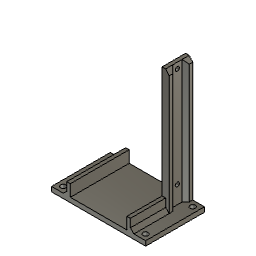
NUC_Mount (Autodesk Fusion 360 design; units mm, degrees)
Autodesk Fusion 360 part; units mm, degrees
sketch "Sketch1" plane through (0, 0, 0) normal (0, 1, 0) x (1, 0, 0)
  line L0 (0, 0) -> (-48, 0) construction
  line L1 (-48, 0) -> (-48, -115) construction
  line L2 (-48, -115) -> (0, -115) construction
  line L3 (0, -115) -> (0, 0) construction
  line L4 (0, -105) -> (3, -105)
  line L5 (3, -105) -> (3, 0)
  line L6 (3, 0) -> (16, 0)
  line L7 (16, 0) -> (16, 4)
  line L8 (16, 4) -> (-64, 4)
  line L9 (-64, 4) -> (-64, 0)
  line L10 (-64, 0) -> (-51, 0)
  line L11 (-51, 0) -> (-51, -10)
  line L12 (-51, -10) -> (-48, -10)
  line L13 (-48, -10) -> (-48, 0)
  line L14 (-48, 0) -> (0, 0)
  line L15 (0, 0) -> (0, -105)
  line L16 (0, -100) -> (3, -100) construction
  line L17 (3, -15) -> (0, -14.9007) construction
  line L18 (-51, 0) -> (-48, 0)
  line L19 (0, 0) -> (3, 0)
  line L20 (3, -105) -> (6, -101.4247)
  line L21 (6, -101.4247) -> (6, 0)
  line L22 (0, -10) -> (3, -10)
  dimension "d1" = 48
  dimension "d2" = 115
  dimension "d3" = 3
  dimension "d4" = 4
  dimension "d6" = 13
  dimension "d7" = 13
  dimension "d8" = 10
  dimension "d9" = 15
  dimension "d10" = 85
  dimension "d11" = 5
  dimension "d16" = 3
  dimension "d17" = 140
  constraint horizontal L0
  constraint vertical L1
  constraint horizontal L2
  constraint vertical L3
  constraint coincident L0.start L3.end
  constraint coincident L3 L4.start
  constraint perpendicular L3 L4
  constraint perpendicular L4 L5
  constraint perpendicular L3 L6
  constraint perpendicular L6 L7
  constraint perpendicular L7 L8
  constraint perpendicular L8 L9
  constraint perpendicular L9 L10
  constraint perpendicular L8 L11
  constraint coincident L1 L12.end
  constraint perpendicular L1 L12
  constraint perpendicular L3 L14
  constraint equal L7 L9
  constraint coincident L3 L16.start
  constraint coincident L5 L16.end
  constraint perpendicular L5 L16
  constraint coincident L5 L17.start
  constraint coincident L3 L17.end
  constraint coincident L6 L0.start
  constraint equal L4 L12
  constraint coincident L5 L4.end
  constraint vertical L21
  constraint coincident L6 L21.end
  constraint coincident L3 L22.start
  constraint coincident L5 L22.end
  constraint perpendicular L5 L22
  constraint collinear L12 L22
  constraint coincident L4.end L5.start
  measures "d1" distance of L0.start L0.end
  measures "d2" distance of L0.end L1.end
  measures "d3" distance of L4.start L4.end
  measures "d4" distance of L6.end L7.end
  measures "d6" distance of L5.end L6.end
  measures "d7" distance of L9.end L10.end
  measures "d8" distance of L10.end L11.end
  measures "d9" vertical distance of L0.start L17.start
  measures "d10" distance of L16.end L17.start
  measures "d11" distance of L4.end L16.end
  measures "d16" distance of L5 L21
  measures "d17" angle of L20 L21
extrude "Extrude1" add sketch "Sketch1" along normal blind 20 contours L4 L5 L15 L22 | L5 L15 L19 L22 | L6 L7 L8 L9 L10 L14 L18 L19 | L11 L12 L13 L18
extrude "Extrude2" add sketch "Sketch1" against normal blind 30 contours L6 L7 L8 L9 L10 L14 L18 L19
extrude "Extrude3" add sketch "Sketch1" against normal blind 30 contours L5 L15 L19 L22 | L11 L12 L13 L18
sketch "Sketch2" plane through (3, 0, 0) normal (1, 0, 0) x (0, 1, 0)
  line L0 (0, 105) -> (0, 10)
  line L1 (0, 10) -> (-30, 10)
  line L2 (-30, 10) -> (-30, 0)
  line L3 (-30, 0) -> (20, 0)
  line L4 (20, 0) -> (20, 105)
  line L5 (20, 105) -> (0, 105)
  line L6 (10, 105) -> (10, 0) construction
  circle A0 centre (10, 15) radius 1.75
  circle A1 centre (10, 100) radius 1.75
  dimension "d21" = 15
  dimension "d22" = 85
  dimension "d23" = 3.5
  constraint midpoint L5 L6.start
  constraint coincident L3 L6.end
  constraint perpendicular L3 L6
  constraint coincident L6 A0.centre
  constraint coincident L6 A1.centre
  constraint equal A0 A1
  measures "d21" distance of L6.end A0.centre
  measures "d22" distance of A0.centre A1.centre
  measures "d23" diameter of A0
extrude "Extrude4" cut sketch "Sketch2" against normal blind 12 contours A0 | A1
extrude "Extrude5" add sketch "Sketch1" along normal blind 3 contours L5 L6 L20 L21
chamfer "Chamfer1" distance 3 angle 45 1 edges at (3, 3, 52.5)
chamfer "Chamfer2" distance 3 angle 45 1 edges at (3, -15, 0)
chamfer "Chamfer3" distance 3 angle 45 1 edges at (-51, -5, 0)
extrude "Extrude6" add sketch "Sketch1" against normal blind 3 from surface at 20 contours L5 L6 L20 L21
chamfer "Chamfer4" distance 3 angle 45 1 edges at (3, 17, 52.5)
sketch "Sketch3" plane through (0, 0, 0) normal (0, 0, 1) x (1, 0, 0)
  line L0 (11, -25) -> (-59, -25) construction
  line L1 (-59, -25) -> (-59, 15) construction
  line L2 (-59, 15) -> (11, 15) construction
  line L3 (11, 15) -> (11, -25) construction
  circle A0 centre (11, -25) radius 2.25
  circle A1 centre (-59, -25) radius 2.25
  circle A2 centre (-59, 15) radius 2.25
  circle A3 centre (11, 15) radius 2.25
  circle A4 centre (11, 15) radius 5 construction
  circle A5 centre (11, -25) radius 5 construction
  circle A6 centre (-59, 15) radius 5 construction
  circle A7 centre (-59, -25) radius 5 construction
  line L4 (-64, -5) -> (20.2305, -5) construction
  line L5 (-64, -30) -> (-64, 20) construction
  line L6 (-24, 20) -> (-24, -32.4373) construction
  line L7 (-48, 20) -> (0, 20) construction
  dimension "d35" = 4.5
  dimension "d36" = 10
  dimension "d37" = 40
  dimension "d38" = 70
  constraint horizontal L0
  constraint vertical L1
  constraint horizontal L2
  constraint vertical L3
  constraint coincident L0.start L3.end
  constraint coincident L0.end L1.start
  constraint coincident L1.end L2.start
  constraint coincident L2.end L3.start
  constraint equal A1 A2
  constraint equal A2 A3
  constraint equal A0 A3
  constraint concentric A3 A4
  constraint concentric A0 A5
  constraint concentric A2 A6
  constraint concentric A1 A7
  constraint equal A5 A6
  constraint equal A5 A7
  constraint equal A4 A7
  constraint perpendicular L3 L4
  constraint coincident L4.start L5
  constraint midpoint L4.start L5
  constraint vertical L6
  constraint coincident L6.start L7
  constraint midpoint L6.start L7
  constraint symmetric L2.end L1.end L6
  constraint symmetric L1.end L0.end L4
  measures "d35" diameter of A1
  measures "d36" diameter of A4
  measures "d37" distance of L0.start L2.end
  measures "d38" distance of L0.start L0.end
extrude "Extrude7" cut sketch "Sketch3" against normal blind 17
equation "d21 = d9"
equation "d22 = d10"
